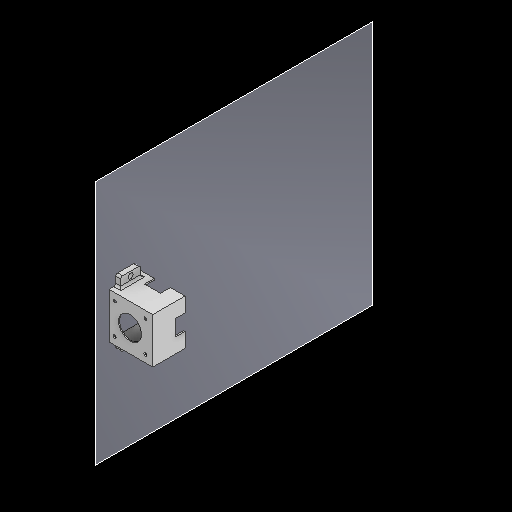
# Autodesk Inventor part: Nema17WheelMotorMountoffset
Saved by Autodesk Inventor 2025 (Build 290162000, 162)
## iProperties
Created: 2024-11-18
Part Number: Nema17WheelMotorMountoffset
Material: Generic
Document SubType Name: Modeling
Designer: Trevor
Density: 1 g/cm^3
Appearance: Default
Author: Trevor
Autodesk Inventor part; units mm, degrees
ref_plane "YZ Plane" through (0, 0, 0) normal (1, 0, 0) x (0, 1, 0)
ref_plane "XZ Plane" through (0, 0, 0) normal (0, 1, 0) x (-1, 0, 0)
sketch "Sketch1" plane through (0, 0, 0) normal (0, 0, 1) x (1, 0, 0)
  line L0 (20.0607, 17.4322) -> (17.4322, 20.0607) construction
  arc A0 (17.4322, 20.0607) -> (16.3716, 20.5) centre (16.3716, 19) ccw construction
  line L1 (16.3716, 20.5) -> (-16.3716, 20.5) construction
  arc A1 (-16.3716, 20.5) -> (-17.4322, 20.0607) centre (-16.3716, 19) ccw construction
  line L2 (-17.4322, 20.0607) -> (-20.0607, 17.4322) construction
  arc A2 (-20.0607, 17.4322) -> (-20.5, 16.3716) centre (-19, 16.3716) ccw construction
  line L3 (-20.5, 16.3716) -> (-20.5, -16.3716) construction
  arc A3 (-20.5, -16.3716) -> (-20.0607, -17.4322) centre (-19, -16.3716) ccw construction
  line L4 (-20.0607, -17.4322) -> (-17.4322, -20.0607) construction
  arc A4 (-17.4322, -20.0607) -> (-16.3716, -20.5) centre (-16.3716, -19) ccw construction
  line L5 (-16.3716, -20.5) -> (16.3716, -20.5) construction
  arc A5 (16.3716, -20.5) -> (17.4322, -20.0607) centre (16.3716, -19) ccw construction
  line L6 (17.4322, -20.0607) -> (20.0607, -17.4322) construction
  arc A6 (20.0607, -17.4322) -> (20.5, -16.3716) centre (19, -16.3716) ccw construction
  line L7 (20.5, -16.3716) -> (20.5, 16.3716) construction
  arc A7 (20.5, 16.3716) -> (20.0607, 17.4322) centre (19, 16.3716) ccw construction
  circle A8 centre (0, 0) radius 16.5 construction
  circle A9 centre (15.5, 15.5) radius 1.55 construction
  circle A10 centre (15.5, -15.5) radius 1.55 construction
  circle A11 centre (-15.5, -15.5) radius 1.55 construction
  circle A12 centre (-15.5, 15.5) radius 1.55 construction
  line L8 (0, 0) -> (-20.3858, 0) construction
  line L9 (-20.3858, 0) -> (-20.3858, -20.3858) construction
  line L10 (-20.3858, -20.3858) -> (0, -20.3858) construction
  line L11 (0, -20.3858) -> (0, 0) construction
  line L12 (0, 0) -> (-20.3858, 0) construction
  line L13 (-20.3858, 0) -> (-20.3858, 20.3858) construction
  line L14 (-20.3858, 20.3858) -> (0, 20.3858) construction
  line L15 (0, 20.3858) -> (0, 0) construction
  line L16 (0, 0) -> (20.3858, 0) construction
  line L17 (20.3858, 0) -> (20.3858, 20.3858) construction
  line L18 (20.3858, 20.3858) -> (0, 20.3858) construction
  line L19 (0, 20.3858) -> (0, 0) construction
  line L20 (0, 0) -> (20.3858, 0) construction
  line L21 (20.3858, 0) -> (20.3858, -20.3858) construction
  line L22 (20.3858, -20.3858) -> (0, -20.3858) construction
  line L23 (0, -20.3858) -> (0, 0) construction
  line L24 (-20.3858, -20.3858) -> (20.3858, -20.3858)
  line L25 (20.3858, -20.3858) -> (20.3858, 20.3858)
  line L26 (20.3858, 20.3858) -> (-20.3858, 20.3858)
  line L27 (-20.3858, 20.3858) -> (-20.3858, -20.3858)
  line L28 (-21.15, -107.4) -> (-21.15, 107.4) projected
  line L29 (-21.15, 22.8858) -> (22.8858, 22.8858)
  line L30 (22.8858, 22.8858) -> (22.8858, -22.8858)
  line L31 (22.8858, -22.8858) -> (-21.15, -22.8858)
  point P0 (0, 0)
  dimension "d0" = 2.5
  constraints: 46 end point, 11 parallel, 6 perpendicular, 5 horizontal, 5 point on line
  measures "d0" distance between parallel lines of L26 L29
ref_plane "Work Plane1" through (-21.15, -21.15, -31.5) normal (0, 0, -1) x (0, 1, 0)
extrude "Extrusion1" add sketch "Sketch1" against normal up to surface (31.5 mm away)
ref_plane "Work Plane2" through (-21.15, -10, -125) normal (1, 0, 0) x (0, 0, 1)
sketch "Sketch2" plane through (-21.15, -10, -125) normal (1, 0, 0) x (0, 0, 1)
  line L0 (125, 12.8858) -> (125, -32.8858) projected
  line L1 (93.5, 12.8858) -> (93.5, -32.8858) projected
  line L2 (125, -32.8858) -> (93.5, -32.8858) projected
  line L3 (125, 12.8858) -> (125, -32.8858) projected
  line L4 (125, 12.8858) -> (93.5, 12.8858) projected
  line L5 (125, -10) -> (93.5, -10) construction
  line L6 (109.25, 12.8858) -> (109.25, -32.8858) construction
  line L7 (109.25, -32.8858) -> (119.25, -32.8858) construction
  line L8 (119.25, -32.8858) -> (119.25, -42.8858)
  line L9 (119.25, -42.8858) -> (109.25, -42.8858)
  line L10 (109.25, -42.8858) -> (109.25, -32.8858) construction
  line L11 (109.25, -42.8858) -> (99.25, -42.8858)
  line L12 (99.25, -42.8858) -> (99.25, -32.8858)
  line L13 (99.25, -32.8858) -> (109.25, -32.8858) construction
  line L14 (109.25, -32.8858) -> (109.25, -42.8858) construction
  line L15 (125, 12.8858) -> (93.5, 12.8858)
  line L16 (119.25, 12.8858) -> (119.25, 22.8858)
  line L17 (119.25, 22.8858) -> (109.25, 22.8858)
  line L18 (109.25, 22.8858) -> (99.25, 22.8858)
  line L19 (99.25, 22.8858) -> (99.25, 12.8858)
  dimension "d3" = 10
  dimension "d4" = 10
  dimension "d5" = 10
  dimension "d6" = 10
  constraints: 30 end point, 6 symmetric about line, 4 parallel, 3 midpoint, 2 horizontal, 2 perpendicular
  measures "d3" distance of L8.end L9.end
  measures "d4" distance of L7.end L8.end
  measures "d5" distance of L12.end L13.end
  measures "d6" distance of L11.end L12.end
extrude "Extrusion2" add sketch "Sketch2" along normal blind 5 contours L4 L19 L18 L17 L16 | L8 L9 L11 L12 L2
sketch "Sketch3" plane through (0, 0, 0) normal (0, 0, 1) x (1, 0, 0)
  line L0 (22.8858, 22.8858) -> (-21.15, 22.8858) projected
  line L1 (-21.15, 22.8858) -> (-21.15, -22.8858) projected
  line L2 (22.8858, 22.8858) -> (-21.15, 22.8858)
  line L3 (-21.15, 22.8858) -> (-21.15, -22.8858)
  line L4 (-21.15, -22.8858) -> (22.8858, -22.8858)
  line L5 (22.8858, -22.8858) -> (22.8858, 22.8858)
  circle A0 centre (-15.5, 15.5) radius 1.25 projected
  circle A1 centre (15.5, 15.5) radius 1.25 projected
  circle A2 centre (-15.5, -15.5) radius 1.25 projected
  circle A3 centre (15.5, -15.5) radius 1.25 projected
  circle A4 centre (0, 0) radius 11 projected
  point P0 (0, 0)
  constraints: 8 end point, 2 parallel, 1 horizontal, 1 perpendicular
extrude "Extrusion3" add sketch "Sketch3" along normal blind 1
fillet "Fillet1" radius 2 10 edges at (-18.65, 22.8858, -25.75) (-18.65, 32.8858, -25.75) (-18.65, 32.8858, -5.75) (-18.65, 22.8858, -5.75) (-18.65, -22.8858, -25.75) (-18.65, -32.8858, -25.75) (-18.65, -32.8858, -5.75) (-18.65, -22.8858, -5.75) (-16.15, -22.8858, -15.75) (-16.15, 22.8858, -15.75)
sketch "Sketch4" plane through (-16.15, -10, -125) normal (1, 0, 0) x (0, 0, -1)
  arc A0 (-117.25, 42.8858) -> (-119.25, 40.8858) centre (-117.25, 40.8858) ccw projected
  line L0 (-119.25, 40.8858) -> (-119.25, 34.8858) projected
  line L1 (-99.25, 34.8858) -> (-119.25, 34.8858) projected
  line L2 (-99.25, 34.8858) -> (-99.25, 40.8858) projected
  arc A1 (-99.25, 40.8858) -> (-101.25, 42.8858) centre (-101.25, 40.8858) ccw projected
  line L3 (-101.25, 42.8858) -> (-117.25, 42.8858) projected
  arc A2 (-119.25, -20.8858) -> (-117.25, -22.8858) centre (-117.25, -20.8858) ccw projected
  line L4 (-117.25, -22.8858) -> (-101.25, -22.8858) projected
  arc A3 (-101.25, -22.8858) -> (-99.25, -20.8858) centre (-101.25, -20.8858) ccw projected
  line L5 (-99.25, -20.8858) -> (-99.25, -14.8858) projected
  line L6 (-119.25, -14.8858) -> (-99.25, -14.8858) projected
  line L7 (-119.25, -14.8858) -> (-119.25, -20.8858) projected
  circle A4 centre (-109.25, 38.7448) radius 2.5
  line L8 (-215.88, 9.0017) -> (215.88, 9.0017) construction
  line L9 (-126, 32.8858) -> (-126, -12.8858) construction
  line L10 (-126, 10) -> (-93.5, 10) construction
  line L11 (-93.5, 32.8858) -> (-93.5, -12.8858) construction
  circle A5 centre (-109.25, -18.7448) radius 2.5
  point P0 (-125, 10)
  dimension "d12" = 5
  constraints: 4 end point, 2 centre point, 2 midpoint, 1 horizontal, 1 symmetric about line, 3 other
  measures "d12" diameter of A4
extrude "Extrusion4" cut sketch "Sketch4" against normal up to surface (5 mm away) contours A4 | A5
sketch "Sketch5" plane through (0, 0, 0) normal (0, 0, -1) x (-1, 0, 0)
  circle A0 centre (0, 0) radius 11 projected
  circle A1 centre (0, 0) radius 11.5
  point P0 (0, 0)
  dimension "d15" = 0.5
  constraints: 1 centre point
  measures "d15" radial gap between concentric circles of A0 A1
extrude "Extrusion5" cut sketch "Sketch5" against normal up to surface (1 mm away) contours A0 | A1
sketch "Sketch6" plane through (22.8858, 22.8858, -31.5) normal (0, 0, -1) x (-1, 0, 0)
  line L0 (43.2716, -2.5) -> (2.5, -2.5) projected
  line L1 (43.2716, -43.2716) -> (43.2716, -2.5) projected
  line L2 (2.5, -43.2716) -> (43.2716, -43.2716) projected
  line L3 (2.5, -2.5) -> (2.5, -43.2716) projected
  line L4 (44.0358, 0) -> (44.0358, -45.7716) projected
  line L5 (0, 0) -> (44.0358, 0) projected
  line L6 (0, -45.7716) -> (0, 0) projected
  line L7 (44.0358, -45.7716) -> (0, -45.7716) projected
  line L8 (1.5, -44.2716) -> (44.2716, -44.2716)
  line L9 (44.2716, -44.2716) -> (44.2716, -1.5)
  line L10 (44.2716, -1.5) -> (1.5, -1.5)
  line L11 (1.5, -1.5) -> (1.5, -44.2716)
  line L12 (44.2716, -44.2716) -> (44.0358, -44.2716)
  line L13 (44.2716, -1.5) -> (44.0358, -1.5)
  point P0 (22.8858, -22.8858)
  dimension "d18" = 1
  constraints: 12 end point, 2 perpendicular, 2 point on line, 3 other
  measures "d18" distance between parallel lines of L3 L11
extrude "Extrusion6" cut sketch "Sketch6" against normal up to surface (31.5 mm away) contours L10 L9 L8 L4 | L4 L8 L11 L10
sketch "Sketch7" plane through (22.8858, -22.8858, -31.5) normal (1, 0, 0) x (0, 0, -1)
  line L0 (-10, 30.8858) -> (-10, 14.8858)
  line L1 (-10, 14.8858) -> (0, 14.8858)
  line L2 (0, 30.8858) -> (-10, 30.8858)
  line L3 (0, 1.5) -> (0, 44.2716) projected
  line L4 (-10, 30.8858) -> (0, 22.8858) construction
  line L5 (-10, 14.8858) -> (0, 22.8858) construction
  point P0 (-31.5, 22.8858)
  dimension "d21" = 16
  constraints: 12 end point, 2 point on line, 1 midpoint, 1 parallel, 1 perpendicular
  measures "d21" distance of L0.start L0.end
extrude "Extrusion7" cut sketch "Sketch7" against normal up to surface (1.5 mm away)
sketch "Sketch8" plane through (-21.15, 22.8858, -31.5) normal (0, 1, 0) x (1, 0, 0)
  line L0 (29.2679, 0) -> (29.2679, -10)
  line L1 (29.2679, -10) -> (13.2679, -10)
  line L2 (13.2679, -10) -> (13.2679, 0)
  line L3 (42.5358, 0) -> (0, 0) projected
  line L4 (21.2679, 0) -> (29.2679, -10) construction
  line L5 (21.2679, 0) -> (13.2679, -10) construction
  point P0 (21.15, -31.5)
  constraints: 12 end point, 2 midpoint, 2 point on line, 1 parallel
extrude "Extrusion8" cut sketch "Sketch8" against normal up to surface (45.7716 mm away)
sketch "Sketch9" plane through (0, 0, 1) normal (0, 0, 1) x (1, 0, 0)
  circle A0 centre (0, 0) radius 11.5 projected
  line L0 (22.8858, 22.8858) -> (-21.15, 22.8858) projected
  line L1 (-21.15, 22.8858) -> (-21.15, -22.8858) projected
  line L2 (-21.15, -22.8858) -> (22.8858, -22.8858) projected
  line L3 (22.8858, -22.8858) -> (22.8858, 22.8858) projected
  circle A1 centre (15.5, -15.5) radius 1.25 projected
  circle A2 centre (-15.5, -15.5) radius 1.25 projected
  circle A3 centre (15.5, 15.5) radius 1.25 projected
  circle A4 centre (-15.5, 15.5) radius 1.25 projected
  circle A5 centre (-15.5, 15.5) radius 1.5
  circle A6 centre (15.5, 15.5) radius 1.5
  circle A7 centre (15.5, -15.5) radius 1.5
  circle A8 centre (-15.5, -15.5) radius 1.5
  point P0 (0, 0)
  dimension "d29" = 0.25
  dimension "d30" = 0.25
  dimension "d31" = 0.25
  dimension "d32" = 0.25
  constraints: 4 centre point
  measures "d29" radial gap between concentric circles of A4 A5
  measures "d30" radial gap between concentric circles of A3 A6
  measures "d31" radial gap between concentric circles of A1 A7
  measures "d32" radial gap between concentric circles of A2 A8
extrude "Extrusion9" cut sketch "Sketch9" against normal up to surface (1 mm away) contours A1 | A2 | A3 | A5 | A6 | A7 | A8
body "Solid1"
